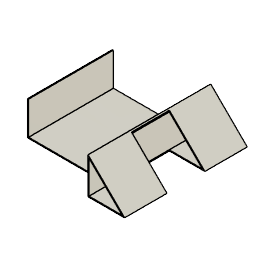
Aluminium Body (Autodesk Fusion 360 design; units mm, degrees)
Autodesk Fusion 360 part; units mm, degrees
sketch "Sketch1" plane through (0, 0, 0) normal (0, 1, 0) x (1, 0, 0)
  line L0 (0, 0) -> (-2, 0)
  line L1 (-2, 0) -> (-2, -72)
  line L2 (-2, -72) -> (0, -72)
  line L3 (0, -72) -> (0, 0)
  line L4 (0, 0) -> (166, 0)
  line L5 (166, 0) -> (166, -2)
  line L6 (166, -2) -> (0, -2)
  line L7 (0, -2) -> (0, 0)
  line L8 (166, -72.909) -> (166, 4.011)
  line L9 (166, -72.909) -> (243.52, 4.011)
  line L10 (166, 4.011) -> (243.52, 4.011)
  line L11 (168, -68.107) -> (238.6649, 2.011)
  line L12 (168, 2.011) -> (238.6649, 2.011)
  line L13 (168, -68.107) -> (168, 2.011)
  dimension "d1" = 2
  dimension "d2" = 72
  dimension "d3" = 166
  dimension "d4" = 2
  dimension "d5" = 76.92
  dimension "d6" = 4.011
  dimension "d8" = 77.52
  dimension "d9" = 2
  constraint horizontal L0
  constraint vertical L1
  constraint horizontal L2
  constraint vertical L3
  constraint coincident L0.start L3.end
  constraint horizontal L4
  constraint vertical L5
  constraint horizontal L6
  constraint vertical L7
  constraint perpendicular L6 L8
  constraint collinear L5 L8
  constraint horizontal L10
  measures "d1" distance of L1.end L2.end
  measures "d2" distance of L0.end L1.end
  measures "d3" distance of L0.start L4.end
  measures "d4" distance of L4.end L5.end
  measures "d5" distance of L8.start L8.end
  measures "d6" distance of L4 L8.end
  measures "d8" horizontal distance of L8.end L9.end
extrude "Extrude1" add sketch "Sketch1" along normal blind 260
sketch "Sketch2" plane through (0, 0, 2) normal (0, 0, 1) x (-1, 0, 0)
  line L0 (0, 0) -> (-166, 0)
  line L1 (-166, 0) -> (-166, -260)
  line L2 (-166, -260) -> (0, -260)
  line L3 (0, -260) -> (0, 0)
  line L4 (2, 0) -> (-166, 0)
  line L5 (-166, 0) -> (-166, -40)
  line L6 (-166, -40) -> (2, -40)
  line L7 (2, -40) -> (2, 0)
  line L8 (0, -130) -> (-166, -130) construction
  line L9 (2, -220) -> (2, -260)
  line L10 (-166, -220) -> (2, -220)
  line L11 (2, -260) -> (-166, -260)
  line L12 (-166, -260) -> (-166, -220)
  point P0 (2, 0)
  dimension "d12" = 168
  dimension "d13" = 40
  constraint horizontal L4
  constraint vertical L5
  constraint horizontal L6
  constraint vertical L7
  constraint coincident L7 P0
  constraint coincident L4 P0
  constraint midpoint L1 L8.end
  constraint midpoint L3 L8.start
  constraint symmetric P0 L8 L9.end
  constraint symmetric L0.end L8 L1.end
  constraint symmetric L5.end L8 L10.start
  constraint symmetric L6.end L8 L9.start
  measures "d12" distance of L5.end L6.end
  measures "d13" distance of L0.end L5.end
extrude "Extrude2" cut sketch "Sketch2" against normal blind 45 contours L0 L1 L3 L4 L5 L6 | L3 L4 L6 L7 | L3 L9 L10 L11 | L1 L2 L3 L10 L11 L12
extrude "Extrude3" cut sketch "Sketch2" along normal blind 80 contours L3 L4 L6 L7 | L3 L9 L10 L11
sketch "Sketch3" plane through (0, 0, 2) normal (0, 0, 1) x (-1, 0, 0)
  line L0 (-166, -220) -> (0, -220)
  line L1 (0, -220) -> (0, -40)
  line L2 (0, -40) -> (-166, -40)
  line L3 (-166, -40) -> (-166, -220)
  line L4 (-168.32, -170) -> (-243.52, -170)
  line L5 (-243.52, -170) -> (-243.52, -90)
  line L6 (-243.52, -90) -> (-168.32, -90)
  line L7 (-168.32, -90) -> (-168.32, -170)
  line L8 (-243.52, 0) -> (-243.52, -260)
  dimension "d18" = 75.2
  dimension "d19" = 80
  constraint horizontal L4
  constraint vertical L5
  constraint horizontal L6
  constraint vertical L7
  constraint coincident L4.end L8
  constraint midpoint L5 L8
  measures "d18" distance of L4.start L4.end
  measures "d19" distance of L4.end L5.end
extrude "Extrude4" cut sketch "Sketch3" along normal mid plane 260 contours L4 L5 L6 L7 L8
equation "d2 = ( 7.2 * 10 ) * 1 mm"
equation "d3 = ( 16.6 * 10 ) * 1 mm"
